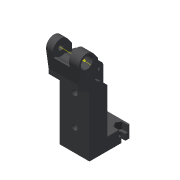
# Autodesk Inventor part: linact_knuckle
Saved by Autodesk Inventor 2014 (Build 180170000, 170)
## iProperties
Created: 2015-04-19
Part Number: linact_knuckle
Material: Generic
Document SubType Name: Modeling
Designer: Martin
Density: 1 g/cm^3
Appearance: Default
Author: Martin
Autodesk Inventor part; units mm, degrees
ref_plane "plane_rodchannel_top" through (-7.5, 5.2285, 6.3) normal (0, 1, 0) x (1, 0, 0)
ref_plane "plane_support_base" through (-7.5, -3.5842, 0) normal (-1, 0, 0) x (0, 0, 1)
sketch "Sketch1" plane through (0, 0, 0) normal (0, 0, 1) x (1, 0, 0)
  circle A0 centre (-0.1255, -7.0715) radius 1 projected
  circle A1 centre (-5.6953, -4.5842) radius 1 projected
  circle A2 centre (5.8715, 6.6985) radius 1 projected
  line L0 (-4.1255, -10.2715) -> (3.8745, -10.2715) projected
  line L1 (-10.5, 0) -> (10.5, 0) projected
  line L2 (0, -14.2715) -> (0, 13.7285) projected
  line L3 (-7.5, -10.2715) -> (7.5, -10.2715)
  line L4 (7.5, -10.2715) -> (7.5, 9.7285)
  line L5 (7.5, 9.7285) -> (-7.5, 9.7285)
  line L6 (-7.5, 9.7285) -> (-7.5, -10.2715)
  line L7 (-7.5, -10.2715) -> (7.5, 9.7285) construction
  line L8 (7.5, -10.2715) -> (-7.5, 9.7285) construction
  circle A3 centre (-0.1255, 1.9285) radius 5.25 projected
  circle A4 centre (-0.1255, 1.9285) radius 5.5
  line L9 (7.5, 7.6985) -> (5.8715, 7.6985)
  line L10 (7.5, 5.6985) -> (5.8715, 5.6985)
  arc A5 (5.8715, 7.6985) -> (5.8715, 5.6985) centre (5.8715, 6.6985) ccw
  line L11 (-5.6953, -5.5842) -> (-7.5, -5.5842)
  line L12 (-5.6953, -3.5842) -> (-7.5, -3.5842)
  arc A6 (-5.6953, -5.5842) -> (-5.6953, -3.5842) centre (-5.6953, -4.5842) ccw
  point P0 (0, 0)
  point P1 (0, -0.2715)
  dimension "d0" = 11
  dimension "d4" = 15
  dimension "d5" = 20
  constraints: 20 end point, 8 point on circle, 8 tangent, 4 parallel, 4 point on line, 3 centre point, 3 midpoint, 3 perpendicular, 1 coincident, 1 collinear, 1 concentric, 1 horizontal
  measures "d0" diameter of A4
  measures "d4" distance of L4.end L5.end
  measures "d5" distance between parallel lines of L0 L5
extrude "ext_base" add sketch "Sketch1" along normal blind 4.3 contours A0 L2 | A0 L2 A4 L1 L4 L3 L0 | L2 A0 | A0 L2 L0 L3 L6 L11 A1 L12 L1 A4 | L1 L6 L5 L2 A4 | A4 L2 L5 L4 L9 A2 L10 L1
sketch "Sketch2" plane through (0, 0, 0) normal (0, 0, -1) x (-1, 0, 0)
  circle A0 centre (0.1255, -7.0715) radius 1 construction
  circle A1 centre (0.1255, -7.0715) radius 1.2
  point P0 (0, 0)
  dimension "d248" = 2.4
  constraints: 1 centre point, 1 coincident
  measures "d248" diameter of A1
extrude "ext_cut_dowel" cut sketch "Sketch2" against normal blind 1
sketch "Sketch3" plane through (0, 0, 4.3) normal (0, 0, 1) x (1, 0, 0)
  circle A0 centre (-0.1255, 1.9285) radius 5.5 projected
  line L0 (-7.5, -10.2715) -> (7.5, -10.2715) projected
  line L1 (7.5, -10.2715) -> (7.5, 5.6985) projected
  line L2 (7.5, 5.6985) -> (5.8715, 5.6985) projected
  arc A1 (5.8715, 7.6985) -> (5.8715, 5.6985) centre (5.8715, 6.6985) ccw projected
  line L3 (5.8715, 7.6985) -> (7.5, 7.6985) projected
  line L4 (7.5, 7.6985) -> (7.5, 9.7285) projected
  line L5 (7.5, 9.7285) -> (-7.5, 9.7285) projected
  line L6 (-7.5, 9.7285) -> (-7.5, -3.5842) projected
  line L7 (-7.5, -3.5842) -> (-5.6953, -3.5842) projected
  arc A2 (-5.6953, -5.5842) -> (-5.6953, -3.5842) centre (-5.6953, -4.5842) ccw projected
  line L8 (-5.6953, -5.5842) -> (-7.5, -5.5842) projected
  line L9 (-7.5, -5.5842) -> (-7.5, -10.2715) projected
  circle A3 centre (-0.1255, 1.9285) radius 3
  line L10 (-7.5, -3.5842) -> (-7.5, -5.5842)
  line L11 (7.5, 7.6985) -> (7.5, 5.6985)
  point P0 (0, 0)
  dimension "d10" = 6
  constraints: 4 end point, 2 collinear, 1 centre point, 1 coincident
  measures "d10" diameter of A3
extrude "ext_bearingstop" add sketch "Sketch3" along normal blind 2 contours A0 | L9 L8 A2 L7 L6 L5 L4 L3 A1 L2 L1 L0 | L10 L7 A2 L8 | L2 A1 L3 L11
sketch "Sketch4" plane through (0, 0, 0) normal (1, 0, 0) x (0, 1, 0)
  line L0 (0, -9.7126) -> (0, 58.2755) projected
  line L1 (-1.0715, 6.3) -> (4.9285, 6.3) projected
  line L2 (-10.2715, 6.3) -> (9.7285, 6.3) projected
  line L3 (9.7285, 6.3) -> (-10.2715, 6.3) projected
  line L4 (-1.0715, 6.3) -> (4.9285, 6.3) projected
  line L5 (1.9285, 6.3) -> (1.9285, 14.2197) construction
  line L6 (-10.2715, 6.3) -> (-1.2715, 6.3)
  line L7 (-1.2715, 6.3) -> (-1.2715, 33.3)
  line L8 (-1.2715, 33.3) -> (-10.2715, 33.3)
  line L9 (-10.2715, 33.3) -> (-10.2715, 6.3)
  line L10 (-10.2715, 6.3) -> (9.7285, 6.3) projected
  line L11 (-1.2715, 13.3) -> (5.7285, 6.3)
  line L12 (5.7285, 6.3) -> (-1.2715, 6.3)
  circle A0 centre (-4.0215, 36.05) radius 1
  circle A1 centre (-13.0215, 45.05) radius 1
  circle A2 centre (-13.0215, 45.05) radius 2.75 construction
  circle A3 centre (-4.0215, 36.05) radius 2.75 construction
  line L13 (-4.0215, 36.05) -> (-13.0215, 36.05) construction
  line L14 (-13.0215, 36.05) -> (-13.0215, 45.05) construction
  line L15 (-1.2715, 33.3) -> (-1.2715, 36.05)
  line L16 (-15.7715, 45.05) -> (-15.7715, 33.3)
  line L17 (-15.7715, 33.3) -> (-10.2715, 30.1246)
  line L18 (-15.7715, 33.3) -> (-10.2715, 33.3) construction
  line L19 (-2.0769, 37.9945) -> (-11.0769, 46.9945)
  arc A4 (-1.2715, 36.05) -> (-2.0769, 37.9945) centre (-4.0215, 36.05) ccw
  arc A5 (-11.0769, 46.9945) -> (-15.7715, 45.05) centre (-13.0215, 45.05) ccw
  point P0 (0, 0)
  point P1 (5.6985, 6)
  point P2 (5.6985, 6)
  point P3 (-3.5842, 6)
  point P4 (-3.5842, 6)
  point P5 (-5.5842, 6)
  point P6 (-5.5842, 6)
  dimension "d13" = 9
  dimension "d17" = 3.2
  dimension "d21" = 45
  dimension "d22" = 7
  dimension "d37" = 27
  dimension "d38" = 2
  dimension "d39" = 5.5
  dimension "d40" = 9
  dimension "d41" = 30
  constraints: 28 end point, 8 point on circle, 7 tangent, 6 centre point, 5 parallel, 4 perpendicular, 3 equal radius, 2 coincident, 2 horizontal, 2 point on line, 1 midpoint, 1 vertical, 2 other
  measures "d13" distance between parallel lines of L9 L7
  measures "d17" distance between parallel lines of L7 L5
  measures "d21" angle of L7 L11
  measures "d22" distance of L11.end L6.end
  measures "d37" distance of L8.end L2.start
  measures "d38" diameter of A1
  measures "d39" diameter of A2
  measures "d40" distance of L13.end L14.end
  measures "d41" angle of L18 L17
extrude "ext_knuckle_column" add sketch "Sketch4" along normal up to surface (15 mm away) from surface at -7.5 contours L7 L2 L9 L8 | L8 L9 L17 L16 A5 L19 A4 L15
ref_plane "plane_basenuts" through (0, 0, 3) normal (0, 0, 1) x (1, 0, 0)
sketch "Sketch8" plane through (0, 0, 3) normal (0, 0, 1) x (1, 0, 0)
  arc A0 (5.8715, 7.6985) -> (5.8715, 5.6985) centre (5.8715, 6.6985) ccw
  arc A1 (-5.6953, -5.5842) -> (-5.6953, -3.5842) centre (-5.6953, -4.5842) ccw
  line L0 (-5.6953, -5.5842) -> (-7, -5.5842)
  line L1 (-7, -5.5842) -> (-7, -10.2715)
  line L2 (-7, -3.2715) -> (-7, -10.2715)
  line L3 (4.6014, 8.8985) -> (3.3312, 6.6985)
  line L4 (3.3312, 6.6985) -> (4.6014, 4.4985)
  line L5 (3.3312, 6.6985) -> (8.4119, 6.6985) construction
  line L6 (4.6014, 8.8985) -> (7.1417, 8.8985)
  line L7 (7.1417, 8.8985) -> (8.4119, 6.6985)
  line L8 (8.4119, 6.6985) -> (7.1417, 4.4985)
  line L9 (4.6014, 4.4985) -> (7.1417, 4.4985)
  line L10 (5.8715, 8.8985) -> (5.8715, 4.4985) construction
  line L11 (0, -14.2715) -> (0, 13.7285)
  line L12 (-8.2357, -4.5842) -> (-3.155, -4.5842) construction
  line L13 (-5.6953, -2.3842) -> (-5.6953, -6.7842) construction
  line L14 (-4.4252, -2.3842) -> (-6.9655, -2.3842)
  line L15 (-6.9655, -2.3842) -> (-8.2357, -4.5842)
  line L16 (-8.2357, -4.5842) -> (-6.9655, -6.7842)
  line L17 (-6.9655, -6.7842) -> (-4.4252, -6.7842)
  line L18 (-4.4252, -6.7842) -> (-3.155, -4.5842)
  line L19 (-4.4252, -2.3842) -> (-3.155, -4.5842)
  line L20 (7.5, -1.2715) -> (7.5, 9.7285) projected
  line L21 (-7.5, 9.7285) -> (-7.5, -1.2715) projected
  line L22 (7.1417, 8.8985) -> (7.5, 8.8985)
  line L23 (7.1417, 4.4985) -> (7.5, 4.4985)
  line L24 (-6.9655, -2.3842) -> (-7.5, -2.3842)
  line L25 (-7.5, -2.3842) -> (-7.5, -6.7842)
  line L26 (-7.5, -6.7842) -> (-6.9655, -6.7842)
  point P0 (0, 0)
  point P1 (-5.7187, -4.5372)
  dimension "d33" = 120
  dimension "d35" = 4.4
  dimension "d36" = 4.4
  constraints: 50 end point, 10 parallel, 8 midpoint, 6 perpendicular, 4 equal length, 4 point on circle, 2 centre point, 2 coincident, 2 point on line, 1 collinear
  measures "d33" angle of L4 L3
  measures "d35" distance between parallel lines of L9 L6
  measures "d36" distance between parallel lines of L17 L14
extrude "ext_cut_basenuts" cut sketch "Sketch8" along normal up to surface (3.3 mm away)
sketch "Sketch9" plane through (-7.5, -10.2715, 0) normal (-1, 0, 0) x (0, 0, 1)
  line L0 (45.05, -5.5) -> (33.3, -5.5) projected
  arc A0 (45.05, -5.5) -> (46.9945, -0.8055) centre (45.05, -2.75) ccw projected
  line L1 (37.9945, 8.1945) -> (46.9945, -0.8055) projected
  arc A1 (37.9945, 8.1945) -> (36.05, 9) centre (36.05, 6.25) ccw projected
  line L2 (6.3, 9) -> (36.05, 9) projected
  circle A2 centre (36.05, 6.25) radius 1 projected
  circle A3 centre (45.05, -2.75) radius 1 projected
  line L3 (29.4109, 9) -> (43.9109, -5.5) construction
  circle A4 centre (36.05, 6.25) radius 2.75 construction
  circle A5 centre (36.05, 6.25) radius 4
  circle A6 centre (45.05, -2.75) radius 4 construction
  line L4 (42.2216, -5.5784) -> (42.1431, -5.5)
  line L5 (42.1431, -5.5) -> (42.1453, -5.5)
  line L6 (28.7038, 9) -> (43.2038, -5.5)
  line L7 (38.55, -8.25) -> (51.55, -8.25)
  line L8 (51.55, -8.25) -> (51.55, 2.75)
  line L9 (51.55, 2.75) -> (38.55, 2.75)
  line L10 (38.55, 2.75) -> (38.55, -8.25)
  line L11 (38.55, -8.25) -> (51.55, 2.75) construction
  line L12 (51.55, -8.25) -> (38.55, 2.75) construction
  point P0 (7, 7)
  point P1 (0, 10.2715)
  point P2 (6, 7)
  dimension "d45" = 8
  dimension "d133" = 0.5
  dimension "d134" = 13
  dimension "d135" = 11
  constraints: 20 end point, 5 parallel, 4 point on line, 3 centre point, 3 coincident, 3 tangent, 2 midpoint, 2 point on circle, 1 equal radius, 1 horizontal, 1 perpendicular, 3 other
  measures "d45" diameter of A5
  measures "d133" distance between parallel lines of L3 L6
  measures "d134" distance of L7.start L7.end
  measures "d135" distance of L7.end L8.end
extrude "ext_cut_finger_right" cut sketch "Sketch9" against normal blind 2
sketch "Sketch11" plane through (-5.5, -10.2715, 0) normal (-1, 0, 0) x (0, 0, 1)
  arc A0 (45.05, -5.5) -> (46.9945, -0.8055) centre (45.05, -2.75) ccw projected
  line L0 (37.9945, 8.1945) -> (46.9945, -0.8055) projected
  arc A1 (37.9945, 8.1945) -> (36.05, 9) centre (36.05, 6.25) ccw projected
  circle A2 centre (45.05, -2.75) radius 1 projected
  circle A3 centre (36.05, 6.25) radius 1 projected
  circle A4 centre (45.05, -2.75) radius 2.75
  circle A5 centre (36.05, 6.25) radius 2.75
  line L1 (42.3, 3.8891) -> (42.3, -2.75) construction
  line L2 (39.7374, 6.4517) -> (42.3937, -3.4618)
  line L3 (39.7374, 6.4517) -> (46.9945, -0.8055)
  line L4 (45.05, -5.5) -> (38.55, -5.5) projected
  line L5 (42.3937, -3.4618) -> (42.3937, -5.5)
  line L6 (42.3937, -5.5) -> (45.05, -5.5)
  circle A6 centre (45.05, -2.75) radius 3.75
  point P0 (0, 10.2715)
  dimension "d47" = 15
  dimension "d136" = 1
  constraints: 10 end point, 6 tangent, 3 centre point, 3 coincident, 3 point on circle, 3 point on line, 1 collinear, 1 concentric, 1 perpendicular, 1 vertical
  measures "d47" angle of L1 L2
  measures "d136" radial gap between concentric circles of A0 A6
extrude "ext_cut_linkattachment" cut sketch "Sketch11" against normal blind 5.5 contours A4 A0 | L4 A6 L5 A4 | A0 L0 A6 L4 | L2 A6 L0 A4 | L5 A6 L2 | L4 L5 A6 | L2 L0 A6
sketch "sk_cut_finger_left" plane through (7.5, -10.2715, 0) normal (1, 0, 0) x (0, 0, -1)
  line L0 (-32.103, 5.6008) -> (-28.7038, 9) projected
  arc A0 (-35.4008, 2.303) -> (-32.103, 5.6008) centre (-36.05, 6.25) ccw projected
  line L1 (-51.55, -8.25) -> (-38.55, -8.25)
  line L2 (-38.55, -8.25) -> (-38.55, 2.75)
  line L3 (-38.55, 2.75) -> (-51.55, 2.75)
  line L4 (-51.55, 2.75) -> (-51.55, -8.25)
  line L5 (-51.55, -8.25) -> (-38.55, 2.75) construction
  line L6 (-38.55, -8.25) -> (-51.55, 2.75) construction
  line L7 (-38.55, 2.75) -> (-34.1135, 2.75)
  arc A1 (-36.05, 9) -> (-37.9945, 8.1945) centre (-36.05, 6.25) ccw projected
  line L8 (-46.9945, -0.8055) -> (-37.9945, 8.1945) projected
  line L9 (-28.7038, 9) -> (-32.103, 5.6008)
  arc A2 (-34.1135, 2.75) -> (-32.103, 5.6008) centre (-36.05, 6.25) ccw
  arc A3 (-46.9945, -0.8055) -> (-45.05, -5.5) centre (-45.05, -2.75) ccw projected
  line L10 (-45.05, -2.75) -> (-38.55, -2.75) construction
  line L11 (-40.05, -4) -> (-38.55, -4)
  line L12 (-38.55, -4) -> (-38.55, -1.5)
  line L13 (-38.55, -1.5) -> (-40.05, -1.5)
  line L14 (-40.05, -1.5) -> (-40.05, -4)
  line L15 (-40.05, -4) -> (-38.55, -1.5) construction
  line L16 (-38.55, -4) -> (-40.05, -1.5) construction
  line L17 (-3, 15.97) -> (-3, 14.77) projected
  line L18 (-51.55, 2.75) -> (-51.55, 9)
  line L19 (-36.05, 9) -> (-6.3, 9) projected
  line L20 (-51.55, 9) -> (-28.7038, 9)
  line L21 (-33.3, -5.5) -> (-45.05, -5.5) projected
  line L22 (-38.55, -5.5) -> (-45.05, -5.5)
  line L23 (-43.4391, 2.75) -> (-46.9945, -0.8055)
  arc A4 (-46.9945, -0.8055) -> (-45.05, -5.5) centre (-45.05, -2.75) ccw
  circle A5 centre (-45.05, -2.75) radius 1 projected
  circle A6 centre (-45.05, -2.75) radius 1
  point P0 (-39.3, -2.75)
  dimension "d137" = 13
  dimension "d138" = 11
  dimension "d149" = 2.5
  dimension "d150" = 1.5
  constraints: 38 end point, 6 parallel, 6 point on circle, 6 point on line, 5 midpoint, 4 perpendicular, 3 centre point, 3 tangent, 2 concentric, 2 horizontal, 1 coincident, 1 collinear
  measures "d137" distance of L1.start L1.end
  measures "d138" distance of L3.end L1.start
  measures "d149" distance of L13.end L11.start
  measures "d150" distance of L11.start L11.end
sketch "sk_squarepot_shaft_reinf" plane through (0, -10.2715, 0) normal (-1, 0, 0) x (0, 0, 1)
  circle A0 centre (45.05, -2.75) radius 1 projected
  line L0 (39.7374, 6.4517) -> (46.9945, -0.8055) projected
  circle A1 centre (45.05, -2.75) radius 3
  circle A2 centre (45.05, -2.75) radius 4
  line L1 (-10.0455, 10.2715) -> (60.273, 10.2715) projected
  arc A3 (44.4933, -6.7111) -> (47.4573, 0.4445) centre (45.05, -2.75) ccw
  line L2 (42.3937, -5.5) -> (42.3937, -5.397) projected
  line L3 (42.1453, -5.5) -> (35.8761, -5.5)
  line L4 (35.8761, -5.5) -> (44.4933, -6.7111)
  line L5 (44.9406, 1.2485) -> (40.5076, 5.6815)
  line L6 (40.5076, 5.6815) -> (47.4573, 0.4445)
  line L7 (45.05, -5.5) -> (42.3937, -5.5) projected
  line L8 (43.4391, 2.75) -> (44.3978, 2.75)
  point P0 (0, 10.2715)
  dimension "d159" = 6
  dimension "d160" = 8
  dimension "d165" = 8
  dimension "d166" = 8
  dimension "d169" = 5.5
  constraints: 10 end point, 9 point on circle, 3 centre point, 3 point on line, 2 coincident, 2 collinear, 2 parallel, 2 tangent, 1 perpendicular
  measures "d159" diameter of A1
  measures "d160" diameter of A2
  measures "d165" angle of L5 L6
  measures "d166" angle of L4 L3
  measures "d169" distance from line of A3.centre L8
extrude "ext_cut_squarepot_shaft" cut sketch "sk_squarepot_shaft_reinf" against normal through all contours A1
extrude "ext_squarepot_reinforcement" add sketch "sk_squarepot_shaft_reinf" against normal up to surface (7.5 mm away) contours L6 L8 L0 | L8 L6 A2 L0 | A2 | A2 L4 L3
extrude "ext_cut_finger_left" cut sketch "sk_cut_finger_left" against normal blind 2 and the other way blind 5 contours A0 L7 L3 L8 A1 L19 L0 | A1 L8 L3 L18 L20
sketch "Sketch33" plane through (0, -10.2715, 0) normal (-1, 0, 0) x (0, 0, 1)
  circle A0 centre (45.05, -2.75) radius 3 projected
  arc A1 (41.7338, -0.9991) -> (42.3937, -5.397) centre (45.05, -2.75) ccw projected
  circle A2 centre (45.05, -2.75) radius 3.75
  line L0 (47.4573, 0.4445) -> (40.5076, 5.6815) projected
  line L1 (50.8, -10.25) -> (45.05, -10.25)
  line L2 (45.05, -10.25) -> (45.05, 4.75)
  line L3 (45.05, 4.75) -> (50.8, 4.75)
  line L4 (50.8, 4.75) -> (50.8, -10.25)
  line L5 (50.8, -10.25) -> (45.05, 4.75) construction
  line L6 (45.05, -10.25) -> (50.8, 4.75) construction
  line L7 (42.3937, -5.397) -> (45.05, -5.397)
  line L8 (45.05, -5.397) -> (45.05, -10.25)
  line L9 (45.05, -10.25) -> (42.3937, -10.25)
  line L10 (42.3937, -10.25) -> (42.3937, -5.397)
  point P0 (0, 10.2715)
  point P1 (47.925, -2.75)
  dimension "d170" = 15
  dimension "d171" = 2
  constraints: 20 end point, 4 parallel, 3 midpoint, 2 coincident, 2 horizontal, 2 perpendicular, 1 centre point, 1 concentric
  measures "d170" distance of L3.end L1.start
  measures "d171" distance edge to line of A2 L4
extrude "ext_cut_link_intrusion" cut sketch "Sketch33" against normal blind 4 contours A0 L2 A2 | A0 L7 A1 A2 L2 | L2 A2 L7 A0 | A0 L7 L2 | L2 L3 L4 L1 A2 | L2 L9 L10 A2 picked at (44.2585, -5.4618)
sketch "Sketch34" plane through (-7.5, -3.5842, 0) normal (-1, 0, 0) x (0, 0, 1)
  line L0 (38.55, -12.1873) -> (38.55, -7.5335) projected
  line L1 (38.55, -7.5335) -> (35.4008, -4.3842) projected
  line L2 (35.8761, -12.1873) -> (44.4933, -13.3983) projected
  arc A0 (44.4933, -13.3983) -> (47.4573, -6.2427) centre (45.05, -9.4373) ccw projected
  line L3 (44.3978, -3.9373) -> (40.5076, -1.0058) projected
  line L4 (47.4573, -6.2427) -> (44.3978, -3.9373)
  line L5 (35.8761, -12.1873) -> (44.4933, -13.3983)
  arc A1 (44.4933, -13.3983) -> (47.4573, -6.2427) centre (45.05, -9.4373) ccw
  circle A2 centre (45.05, -9.4373) radius 1.25
  line L6 (44.3978, -3.9373) -> (33.3, -3.9373)
  line L7 (33.3, -3.9373) -> (33.3, -12.1873)
  line L8 (33.3, -12.1873) -> (35.8761, -12.1873)
  point P0 (45.05, -9.4373)
  dimension "d174" = 2.5
  dimension "d176" = 5.5
  constraints: 10 end point, 2 centre point, 2 perpendicular, 2 point on circle, 2 tangent, 1 coincident, 1 collinear, 1 parallel, 1 point on line
  measures "d174" diameter of A2
  measures "d176" distance from line of A0.centre L6
extrude "ext_link_reinforcement" add sketch "Sketch34" against normal up to surface (2 mm away)
sketch "sk_potbody" plane through (7.5, -10.2715, 0) normal (1, 0, 0) x (0, 0, -1)
  arc A0 (-47.4573, 0.4445) -> (-44.4933, -6.7111) centre (-45.05, -2.75) ccw projected
  circle A1 centre (-45.05, -2.75) radius 3 projected
  line L0 (-38.55, -8.25) -> (-51.55, -8.25) construction
  line L1 (-51.55, -8.25) -> (-51.55, 2.75) construction
  line L2 (-51.55, 2.75) -> (-38.55, 2.75) construction
  line L3 (-38.55, 2.75) -> (-38.55, -8.25)
  line L4 (-38.55, -8.25) -> (-51.55, 2.75) construction
  line L5 (-51.55, -8.25) -> (-38.55, 2.75) construction
  line L6 (-47.4573, 0.4445) -> (-44.3978, 2.75) projected
  line L7 (-35.8761, -5.5) -> (-44.4933, -6.7111) projected
  line L8 (-45.05, -2.75) -> (-38.55, -2.75) construction
  line L9 (-40.05, -4) -> (-38.55, -4)
  line L10 (-38.55, -4) -> (-38.55, -1.5)
  line L11 (-38.55, -1.5) -> (-40.05, -1.5)
  line L12 (-40.05, -1.5) -> (-40.05, -4)
  line L13 (-40.05, -4) -> (-38.55, -1.5) construction
  line L14 (-38.55, -4) -> (-40.05, -1.5) construction
  line L15 (-44.3978, 2.75) -> (-47.4573, 0.4445)
  line L16 (-44.4933, -6.7111) -> (-38.55, -5.8758)
  arc A2 (-47.4573, 0.4445) -> (-44.4933, -6.7111) centre (-45.05, -2.75) ccw
  circle A3 centre (-45.05, -2.75) radius 3
  line L17 (-38.55, 2.75) -> (-44.3978, 2.75)
  point P0 (-39.3, -2.75)
  point P1 (-39.3, -2.75)
  dimension "d223" = 11
  dimension "d224" = 13
  dimension "d225" = 2.5
  dimension "d226" = 1.5
  constraints: 32 end point, 6 midpoint, 5 equal length, 4 point on line, 2 centre point, 2 horizontal, 2 perpendicular, 2 point on circle, 2 tangent, 1 coincident, 1 concentric
  measures "d223" distance of L0.end L1.end
  measures "d224" distance of L0.start L0.end
  measures "d225" distance of L11.end L9.start
  measures "d226" distance of L9.start L9.end
extrude "ext_squarepot_body" add sketch "sk_potbody" along normal blind 1.5 contours L6 L17 L3 L11 L12 L9 L7 A0
extrude "ext_cut_squarepot_tab" cut sketch "sk_potbody" against normal blind 1.5 contours L9 L12 L11 L3
sketch "Sketch42" plane through (0, -10.2715, 0) normal (-1, 0, 0) x (0, 0, 1)
  line L0 (42.3937, -6.416) -> (42.3937, -5.5) projected
  line L1 (35.8761, -5.5) -> (42.3937, -5.5) projected
  line L2 (35.8761, -5.5) -> (42.3937, -6.416) projected
  point P0 (0, 10.2715)
extrude "QFIX_ext_backdetail" add sketch "Sketch42" along normal up to surface (5.5 mm away)
sketch "Sketch45" plane through (-5.5, -16.6875, 42.3937) normal (1, 0, 0) x (0, 0, -1)
  line L0 (0, 0) -> (0, 1.019) projected
  arc A0 (0, 1.019) -> (0.6599, 5.4169) centre (-2.6563, 3.666) ccw projected
  line L1 (0.6599, 5.4169) -> (1.6644, 9.166) projected
  line L2 (-2.0041, 9.166) -> (1.6644, 9.166) projected
  line L3 (-5.0636, 6.8605) -> (-2.0041, 9.166) projected
  arc A1 (-5.0636, 6.8605) -> (-2.0996, -0.2951) centre (-2.6563, 3.666) ccw projected
  line L4 (0, 0) -> (-2.0996, -0.2951) projected
  circle A2 centre (-2.6563, 3.666) radius 1.25 projected
  point P0 (42.3937, 16.6875)
extrude "QFIX_ext_link_reinforcemet_extrathick" add sketch "Sketch45" along normal blind 1.5
sketch "Sketch46" plane through (0, -10.2715, 0) normal (-1, 0, 0) x (0, 0, 1)
  arc A0 (45.05, 1) -> (41.7338, -0.9991) centre (45.05, -2.75) ccw projected
  line L0 (45.05, 1) -> (45.05, 2.2585) projected
  line L1 (45.05, 2.2585) -> (40.5076, 5.6815) projected
  line L2 (39.7374, 6.4517) -> (40.5076, 5.6815) projected
  line L3 (41.7338, -0.9991) -> (39.7374, 6.4517) projected
  point P0 (0, 10.2715)
extrude "QFIX_ext_link_intrusion_xtraspace" cut sketch "Sketch46" against normal blind 1
sketch "Sketch44" plane through (-7.5, -1.2715, 6.3) normal (0, 1, 0) x (1, 0, 0)
  line L0 (0, 0) -> (15, 0) projected
  line L1 (7.5, 16.11) -> (7.5, -52.56) projected
  circle A0 centre (7.5, -5) radius 1.5
  circle A1 centre (7.5, -20) radius 1.5
  dimension "d238" = 3
  dimension "d239" = 15
  dimension "d240" = 5
  constraints: 2 centre point, 2 point on line, 1 equal radius
  measures "d238" diameter of A0
  measures "d239" distance of A1.centre A0.centre
  measures "d240" distance from line of L0 A0.centre
extrude "ext_cut_mountingholes" cut sketch "Sketch44" against normal through all
sketch "sk_support_base_1" plane through (-7.5, -3.5842, 0) normal (-1, 0, 0) x (0, 0, 1)
  line L0 (28.7038, 2.3127) -> (36.05, 2.3127) projected
  line L1 (44.3978, -3.9373) -> (34.1135, -3.9373) projected
  line L2 (32.103, -1.0865) -> (28.7038, 2.3127) projected
  line L3 (30.118, 2.3127) -> (35.368, -2.9373)
  line L4 (35.368, -2.9373) -> (45.368, -2.9373)
  line L5 (45.368, -2.9373) -> (40.118, 2.3127)
  line L6 (40.118, 2.3127) -> (30.118, 2.3127)
  point P0 (0, 3.5842)
  dimension "d187" = 1
  dimension "d188" = 1
  dimension "d189" = 10
  dimension "d194" = 1
  dimension "d196" = 1
  dimension "d197" = 1
  dimension "d200" = 1
  constraints: 22 end point, 6 point on circle, 3 parallel, 3 point on line, 2 centre point, 1 coincident, 1 tangent
  measures "d196" distance between parallel lines of L1 L0
equation "\"d0\" = linact_bearing_diameter"
equation "\"d4\" = model_column_thickness"
equation "\"d6\" = linact_bearing_thickness"
equation "\"d39\" = general_bore_smallersupport_diameter"
equation "\"d42\" = -0.5 * model_fingerbase_thickness + 0.5 * model_column_thickness"
equation "\"general_bore_smallersupport_diameter\" = 5.5"
equation "\"model_column_thickness\" = 15"
equation "\"model_fingerbase_thickness\" = 11"
equation "\"linact_bearing_diameter\" = 11"
equation "\"linact_bearing_thickness\" = 4.3"
body "Solid1"
